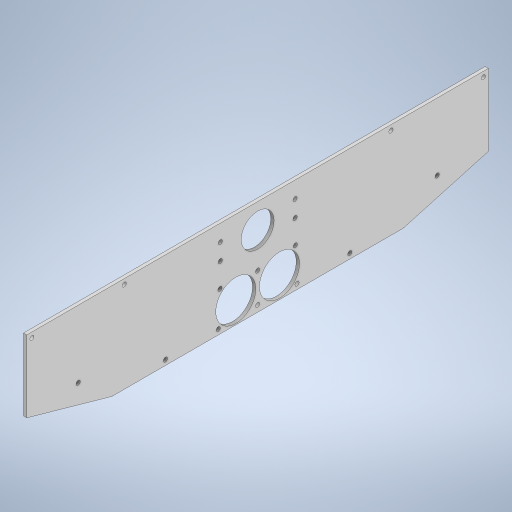
# Autodesk Inventor part: insideChassiPlate2.0
Saved by Autodesk Inventor 2023 (Build 270158000, 158)
## iProperties
Created: 2022-09-08
Part Number: insideChassiPlate2.0
Material: Generic
Document SubType Name: Modeling
Designer: deli
Density: 1 g/cm^3
Appearance: Default
Author: deli
Autodesk Inventor part; units mm, degrees
ref_plane "YZ Plane" through (0, 0, 0) normal (1, 0, 0) x (0, 1, 0)
ref_plane "XZ Plane" through (0, 0, 0) normal (0, 1, 0) x (-1, 0, 0)
ref_plane "XY Plane" through (0, 0, 0) normal (0, 0, 1) x (1, 0, 0)
sketch "Sketch1" plane through (0, 0, 0) normal (1, 0, 0) x (0, 1, 0)
  line L0 (-34.0027, 86.5738) -> (-104.0027, 86.5738) projected
  line L1 (-104.0027, 86.5738) -> (-127.2253, 4.3058) projected
  arc A0 (-127.2253, 4.3058) -> (-127.4133, 2.9475) centre (-122.4133, 2.9475) ccw projected
  line L2 (-127.4133, 2.9475) -> (-127.4133, -279.7999) projected
  arc A1 (-127.4133, -279.7999) -> (-127.2253, -281.1582) centre (-122.4133, -279.7999) ccw projected
  line L3 (-127.2253, -281.1582) -> (-104.0027, -363.4262) projected
  line L4 (-104.0027, -363.4262) -> (-34.0027, -363.4262) projected
  line L5 (-34.0027, -363.4262) -> (-34.0027, -226.9762) projected
  line L6 (-34.0027, -226.9762) -> (230.9973, -226.9762) projected
  line L7 (230.9973, -226.9762) -> (230.9973, -201.5762) projected
  line L8 (230.9973, -201.5762) -> (-34.0027, -201.5762) projected
  line L9 (-34.0027, -201.5762) -> (-34.0027, 86.5738) projected
  circle A2 centre (-66.0027, -101.9662) radius 2 projected
  circle A3 centre (-122.4133, -228.31) radius 2 projected
  circle A4 centre (-122.4133, -48.5424) radius 2 projected
  circle A5 centre (-39.0027, -8.4262) radius 2 projected
  circle A6 centre (-39.0027, -358.4262) radius 2 projected
  circle A7 centre (-89.2685, -175.1441) radius 2 projected
  circle A8 centre (-99.4133, 36.5738) radius 2 projected
  circle A9 centre (-99.4133, -313.4262) radius 2 projected
  circle A10 centre (-106.6633, -117.135) radius 7 construction
  circle A11 centre (-106.6633, -159.7175) radius 7 construction
  circle A12 centre (-92.1807, -138.4262) radius 2 projected
  circle A13 centre (-121.1459, -138.4262) radius 2 projected
  circle A14 centre (-122.4133, -100.0323) radius 2 projected
  circle A15 centre (-122.4133, -176.8201) radius 2 projected
  circle A16 centre (-39.0027, 81.5738) radius 2 projected
  circle A17 centre (-89.2685, -101.7083) radius 2 projected
  circle A18 centre (-39.0027, -268.4262) radius 2 projected
  circle A19 centre (222.9973, -212.6887) radius 2 projected
  circle A20 centre (-58.0027, -138.4262) radius 16 projected
  circle A21 centre (-50.0027, -101.9662) radius 2 projected
  line L10 (-34.0027, -201.5762) -> (-34.0027, -226.9762)
  spline S0 degree 3 poles (-44.0027, -174.8862) (-44.0027, -175.0973) (-43.9693, -175.3071) (-43.8358, -175.7154) (-43.7344, -175.9104) (-43.4447, -176.2972) (-43.2452, -176.4757) (-42.7979, -176.7388) (-42.5566, -176.8247) (-42.0448, -176.9031) (-41.7788, -176.8911) (-41.2697, -176.7652) (-41.0313, -176.6538) (-40.6137, -176.3479) (-40.4377, -176.1576) (-40.1619, -175.7123) (-40.0681, -175.4594) (-39.9874, -174.9441) (-39.9964, -174.6875) (-40.1114, -174.1861) (-40.2182, -173.9465) (-40.5206, -173.5174) (-40.7149, -173.3332) (-41.1541, -173.0576) (-41.3924, -172.9648) (-41.9003, -172.8716) (-42.1657, -172.8756) (-42.6799, -172.9861) (-42.9235, -173.0914) (-43.3506, -173.3866) (-43.5314, -173.5713) (-43.8189, -174.0074) (-43.9197, -174.2567) (-44.0156, -174.7696) (-44.0141, -175.0274) (-43.9132, -175.5321) (-43.8136, -175.774) (-43.5242, -176.2111) (-43.3354, -176.401) (-42.9045, -176.6892) (-42.6692, -176.7888) (-42.1652, -176.8968) (-41.9006, -176.9007) (-41.3816, -176.8057) (-41.1326, -176.7065) (-40.6963, -176.422) (-40.511, -176.2427) (-40.2122, -175.816) (-40.1048, -175.5704) (-39.9938, -175.0601) (-39.9881, -174.801) (-40.0753, -174.2932) (-40.168, -174.0493) (-40.4445, -173.6047) (-40.6279, -173.4096) (-41.0506, -173.1092) (-41.2831, -173.003) (-41.7833, -172.8812) (-42.047, -172.8697) (-42.5675, -172.9494) (-42.819, -173.0412) (-43.2627, -173.3122) (-43.4527, -173.4853) (-43.7634, -173.9013) (-43.8782, -174.1427) (-44.0055, -174.6501) (-44.0192, -174.9106) (-43.9469, -175.4217) (-43.8618, -175.6674) (-43.5979, -176.122) (-43.4182, -176.3244) (-43.0011, -176.6377) (-42.7711, -176.7501) (-42.2746, -176.8847) (-42.012, -176.9031) (-41.4904, -176.8376) (-41.2366, -176.7526) (-40.7865, -176.4941) (-40.5923, -176.3268) (-40.2708, -175.9206) (-40.1496, -175.6833) (-40.0072, -175.1788) (-39.9861, -174.9169) (-40.0451, -174.403) (-40.1233, -174.1557) (-40.3739, -173.6953) (-40.5474, -173.4886) (-40.9581, -173.1613) (-41.189, -173.0411) (-41.6904, -172.8931) (-41.9568, -172.8693) (-42.4735, -172.9258) (-42.7193, -173.0017) (-43.1803, -173.2476) (-43.3886, -173.4196) (-43.7216, -173.8308) (-43.8448, -174.0644) (-43.9918, -174.5579) (-44.0174, -174.8122) (-43.9712, -175.3286) (-43.8952, -175.5854) (-43.6507, -176.0485) (-43.4868, -176.2516) (-43.0923, -176.5829) (-42.8659, -176.7085) (-42.3694, -176.8702) (-42.103, -176.9013) (-41.5836, -176.8584) (-41.3353, -176.7888) (-40.8699, -176.5556) (-40.659, -176.391) (-40.3152, -175.9912) (-40.185, -175.7606) (-40.0238, -175.2709) (-39.9911, -175.0175) (-40.0225, -174.5) (-40.0911, -174.2412) (-40.3226, -173.7707) (-40.4812, -173.5625) (-40.8661, -173.2209) (-41.0877, -173.0896) (-41.5789, -172.9136) (-41.8451, -172.8747) (-42.3669, -172.903) (-42.6178, -172.966) (-43.0878, -173.1857) (-43.3013, -173.3426) (-43.6561, -173.7305) (-43.7936, -173.9577) (-43.9695, -174.4435) (-44.0097, -174.6961) (-43.9934, -175.2144) (-43.9324, -175.4751) (-43.7145, -175.9528) (-43.5615, -176.166) (-43.1865, -176.5182) (-42.9696, -176.6553) (-42.4841, -176.8457) (-42.2183, -176.8924) (-41.6944, -176.8789) (-41.4411, -176.8229) (-40.9667, -176.6166) (-40.7505, -176.4673) (-40.385, -176.0915) (-40.2403, -175.8678) (-40.0496, -175.3861) (-40.002, -175.1343) (-40.0035, -174.6152) (-40.057, -174.353) (-40.2614, -173.8686) (-40.4087, -173.6505) (-40.7738, -173.2881) (-40.9862, -173.1452) (-41.4662, -172.941) (-41.7314, -172.8867) (-42.2569, -172.8858) (-42.5123, -172.9351) (-42.991, -173.1283) (-43.2096, -173.2706) (-43.5852, -173.6348) (-43.7367, -173.8549) (-43.9413, -174.3322) (-43.996, -174.5833) (-44.0086, -175.103) (-43.9622, -175.3667) (-43.7706, -175.8572) (-43.6287, -176.0797) (-43.2729, -176.4517) (-43.0646, -176.5999) (-42.593, -176.8155) (-42.3322, -176.8766) (-41.809, -176.8935) (-41.5515, -176.8517) (-41.0682, -176.673) (-40.8468, -176.5384) (-40.4604, -176.1869) (-40.3016, -175.9709) (-40.0818, -175.4987) (-40.0193, -175.2486) (-39.9914, -174.7284) (-40.03, -174.4632) (-40.2076, -173.9663) (-40.3435, -173.7392) (-40.6892, -173.3569) (-40.8932, -173.2031) (-41.3584, -172.9744) (-41.6173, -172.9059) (-42.1406, -172.8742) (-42.3998, -172.909) (-42.8872, -173.0743) (-43.1112, -173.202) (-43.5072, -173.5418) (-43.6726, -173.7538) (-43.9062, -174.221) (-43.9757, -174.47) (-44.0174, -174.9874) (-43.9867, -175.2511) (-43.8249, -175.7515) (-43.6955, -175.9833) (-43.3606, -176.3764) (-43.161, -176.5362) (-42.7026, -176.7785) (-42.4458, -176.8544) (-41.923, -176.9014) (-41.6622, -176.8741) (-41.1706, -176.7226) (-40.9439, -176.6019) (-40.5382, -176.2741) (-40.3662, -176.0664) (-40.1187, -175.6048) (-40.0421, -175.3571) (-39.9863, -174.8425) (-40.0091, -174.5803) (-40.155, -174.0766) (-40.2778, -173.8403) (-40.6017, -173.4365) (-40.7969, -173.2705) (-41.2486, -173.015) (-41.5029, -172.9316) (-42.0248, -172.8694) (-42.2871, -172.8895) (-42.7828, -173.0272) (-43.0121, -173.1411) (-43.4272, -173.457) (-43.6055, -173.6603) (-43.8665, -174.1162) (-43.95, -174.3623) (-44.0194, -174.8741) (-44.004, -175.1349) (-43.8734, -175.6416) (-43.7572, -175.8821) (-43.4441, -176.296) (-43.2531, -176.4678) (-42.808, -176.736) (-42.556, -176.8264) (-42.0351, -176.9029) (-41.7717, -176.8899) (-41.2723, -176.7652) (-41.0404, -176.6577) (-40.6194, -176.3548) (-40.4371, -176.1586) (-40.1632, -175.7125) (-40.072, -175.4683) (-39.9876, -174.9599) (-39.9949, -174.7005) (-40.1089, -174.1907) (-40.2178, -173.9459) (-40.5188, -173.5212) (-40.705, -173.3431) (-41.1433, -173.0608) (-41.3933, -172.9628) (-41.9133, -172.8711) (-42.1778, -172.8767) (-42.6809, -172.9877) (-42.9156, -173.0888) (-43.3447, -173.3797) (-43.5324, -173.5707) (-43.8189, -174.0095) (-43.9171, -174.2518) (-44.0149, -174.7572) (-44.0149, -175.0153) (-43.9157, -175.5277) (-43.8135, -175.7762) (-43.5234, -176.2102) (-43.3417, -176.3938) (-42.9126, -176.6866) (-42.6678, -176.7907) (-42.1526, -176.8978) (-41.8873, -176.9001) (-41.3802, -176.8037) (-41.1426, -176.7095) (-40.7052, -176.4311) (-40.512, -176.2456) (-40.2124, -175.8148) (-40.1071, -175.5747) (-39.9952, -175.0726) (-39.9878, -174.8157) (-40.0718, -174.3009) (-40.167, -174.0488) (-40.4398, -173.6142) (-40.6083, -173.4315) (-40.9968, -173.1412) (-41.2121, -173.0337) (-41.4412, -172.9667) knots 0.000001 0.000001 0.000001 0.000001 0.063398 0.063398 0.128915 0.128915 0.208453 0.208453 0.284598 0.284598 0.36365 0.36365 0.441803 0.441803 0.518819 0.518819 0.598884 0.598884 0.675195 0.675195 0.753106 0.753106 0.832585 0.832585 0.908527 0.908527 0.987293 0.987293 1.06607 1.06607 1.142839 1.142839 1.222632 1.222632 1.299213 1.299213 1.376876 1.376876 1.456341 1.456341 1.532212 1.532212 1.610735 1.610735 1.690252 1.690252 1.766822 1.766822 1.846392 1.846392 1.923362 1.923362 2.000828 2.000828 2.080319 2.080319 2.156245 2.156245 2.234575 2.234575 2.31405 2.31405 2.390444 2.390444 2.469816 2.469816 2.547344 2.547344 2.624642 2.624642 2.705021 2.705021 2.781115 2.781115 2.859312 2.859312 2.938796 2.938796 3.01493 3.01493 3.093973 3.093973 3.171944 3.171944 3.248946 3.248946 3.329001 3.329001 3.406279 3.406279 3.485634 3.485634 3.562005 3.562005 3.642108 3.642108 3.720394 3.720394 3.796227 3.796227 3.875634 3.875634 3.953058 3.953058 4.029875 4.029875 4.109405 4.109405 4.185934 4.185934 4.265232 4.265232 4.34372 4.34372 4.419521 4.419521 4.498908 4.498908 4.576539 4.576539 4.652987 4.652987 4.732749 4.732749 4.809486 4.809486 4.888063 4.888063 4.966802 4.966802 5.042698 5.042698 5.122108 5.122108 5.199994 5.199994 5.276196 5.276196 5.356239 5.356239 5.433231 5.433231 5.51121 5.51121 5.590242 5.590242 5.666365 5.666365 5.745842 5.745842 5.824027 5.824027 5.900118 5.900118 5.980485 5.980485 6.057771 6.057771 6.135304 6.135304 6.214664 6.214664 6.291046 6.291046 6.370513 6.370513 6.448831 6.448831 6.524751 6.524751 6.604234 6.604234 6.681689 6.681689 6.758659 6.758659 6.838216 6.838216 6.914774 6.914774 6.994299 6.994299 7.072809 7.072809 7.148671 7.148671 7.228128 7.228128 7.305778 7.305778 7.382357 7.382357 7.462136 7.462136 7.538892 7.538892 7.617675 7.617675 7.696426 7.696426 7.772357 7.772357 7.851827 7.851827 7.929724 7.929724 8.00603 8.00603 8.08608 8.08608 8.163082 8.163082 8.241238 8.241238 8.320275 8.320275 8.396406 8.396406 8.475934 8.475934 8.554121 8.554121 8.630289 8.630289 8.710655 8.710655 8.787944 8.787944 8.865621 8.865621 8.944979 8.944979 9.021361 9.021361 9.100863 9.100863 9.179179 9.179179 9.255149 9.255149 9.334671 9.334671 9.412121 9.412121 9.489205 9.489205 9.568755 9.568755 9.645307 9.645307 9.725014 9.725014 9.803511 9.803511 9.879402 9.879402 9.958888 9.958888 10.036524 10.036524 10.113198 10.113198 10.192958 10.192958 10.269699 10.269699 10.348645 10.348645 10.427375 10.427375 10.503309 10.503309 10.582801 10.582801 10.660674 10.660674 10.737051 10.737051 10.817073 10.817073 10.890944 10.890944 10.962515 10.962515 10.962515 10.962515 projected
  spline S1 degree 3 poles (-76.0027, -174.8862) (-76.0027, -175.0973) (-75.9693, -175.3071) (-75.8358, -175.7154) (-75.7344, -175.9104) (-75.4447, -176.2972) (-75.2452, -176.4757) (-74.7979, -176.7388) (-74.5566, -176.8247) (-74.0448, -176.9031) (-73.7788, -176.8911) (-73.2697, -176.7652) (-73.0313, -176.6538) (-72.6137, -176.3479) (-72.4377, -176.1576) (-72.1619, -175.7123) (-72.0681, -175.4594) (-71.9874, -174.9441) (-71.9964, -174.6875) (-72.1114, -174.1861) (-72.2182, -173.9465) (-72.5206, -173.5174) (-72.7149, -173.3332) (-73.1541, -173.0576) (-73.3924, -172.9648) (-73.9003, -172.8716) (-74.1657, -172.8756) (-74.6799, -172.9861) (-74.9235, -173.0914) (-75.3506, -173.3866) (-75.5314, -173.5713) (-75.8189, -174.0074) (-75.9197, -174.2567) (-76.0156, -174.7696) (-76.0141, -175.0274) (-75.9132, -175.5321) (-75.8136, -175.774) (-75.5242, -176.2111) (-75.3354, -176.401) (-74.9045, -176.6892) (-74.6692, -176.7888) (-74.1652, -176.8968) (-73.9006, -176.9007) (-73.3816, -176.8057) (-73.1326, -176.7065) (-72.6963, -176.422) (-72.511, -176.2427) (-72.2122, -175.816) (-72.1048, -175.5704) (-71.9938, -175.0601) (-71.9881, -174.801) (-72.0753, -174.2932) (-72.168, -174.0493) (-72.4445, -173.6047) (-72.6279, -173.4096) (-73.0506, -173.1092) (-73.2831, -173.003) (-73.7833, -172.8812) (-74.047, -172.8697) (-74.5675, -172.9494) (-74.819, -173.0412) (-75.2627, -173.3122) (-75.4527, -173.4853) (-75.7634, -173.9013) (-75.8782, -174.1427) (-76.0055, -174.6501) (-76.0192, -174.9106) (-75.9469, -175.4217) (-75.8618, -175.6674) (-75.5979, -176.122) (-75.4182, -176.3244) (-75.0011, -176.6377) (-74.7711, -176.7501) (-74.2746, -176.8847) (-74.012, -176.9031) (-73.4904, -176.8376) (-73.2366, -176.7526) (-72.7865, -176.4941) (-72.5923, -176.3268) (-72.2708, -175.9206) (-72.1496, -175.6833) (-72.0072, -175.1788) (-71.9861, -174.9169) (-72.0451, -174.403) (-72.1233, -174.1557) (-72.3739, -173.6953) (-72.5474, -173.4886) (-72.9581, -173.1613) (-73.189, -173.0411) (-73.6904, -172.8931) (-73.9568, -172.8693) (-74.4735, -172.9258) (-74.7193, -173.0017) (-75.1803, -173.2476) (-75.3886, -173.4196) (-75.7216, -173.8308) (-75.8448, -174.0644) (-75.9918, -174.5579) (-76.0174, -174.8122) (-75.9712, -175.3286) (-75.8952, -175.5854) (-75.6507, -176.0485) (-75.4868, -176.2516) (-75.0923, -176.5829) (-74.8659, -176.7085) (-74.3694, -176.8702) (-74.103, -176.9013) (-73.5836, -176.8584) (-73.3353, -176.7888) (-72.8699, -176.5556) (-72.659, -176.391) (-72.3152, -175.9912) (-72.185, -175.7606) (-72.0238, -175.2709) (-71.9911, -175.0175) (-72.0225, -174.5) (-72.0911, -174.2412) (-72.3226, -173.7707) (-72.4812, -173.5625) (-72.8661, -173.2209) (-73.0877, -173.0896) (-73.5789, -172.9136) (-73.8451, -172.8747) (-74.3669, -172.903) (-74.6178, -172.966) (-75.0878, -173.1857) (-75.3013, -173.3426) (-75.6561, -173.7305) (-75.7936, -173.9577) (-75.9695, -174.4435) (-76.0097, -174.6961) (-75.9934, -175.2144) (-75.9324, -175.4751) (-75.7145, -175.9528) (-75.5615, -176.166) (-75.1865, -176.5182) (-74.9696, -176.6553) (-74.4841, -176.8457) (-74.2183, -176.8924) (-73.6944, -176.8789) (-73.4411, -176.8229) (-72.9667, -176.6166) (-72.7505, -176.4673) (-72.385, -176.0915) (-72.2403, -175.8678) (-72.0496, -175.3861) (-72.002, -175.1343) (-72.0035, -174.6152) (-72.057, -174.353) (-72.2614, -173.8686) (-72.4087, -173.6505) (-72.7738, -173.2881) (-72.9862, -173.1452) (-73.4662, -172.941) (-73.7314, -172.8867) (-74.2569, -172.8858) (-74.5123, -172.9351) (-74.991, -173.1283) (-75.2096, -173.2706) (-75.5852, -173.6348) (-75.7367, -173.8549) (-75.9413, -174.3322) (-75.996, -174.5833) (-76.0086, -175.103) (-75.9622, -175.3667) (-75.7706, -175.8572) (-75.6287, -176.0797) (-75.2729, -176.4517) (-75.0646, -176.5999) (-74.593, -176.8155) (-74.3322, -176.8766) (-73.809, -176.8935) (-73.5515, -176.8517) (-73.0682, -176.673) (-72.8468, -176.5384) (-72.4604, -176.1869) (-72.3016, -175.9709) (-72.0818, -175.4987) (-72.0193, -175.2486) (-71.9914, -174.7284) (-72.03, -174.4632) (-72.2076, -173.9663) (-72.3435, -173.7392) (-72.6892, -173.3569) (-72.8932, -173.2031) (-73.3584, -172.9744) (-73.6173, -172.9059) (-74.1406, -172.8742) (-74.3998, -172.909) (-74.8872, -173.0743) (-75.1112, -173.202) (-75.5072, -173.5418) (-75.6726, -173.7538) (-75.9062, -174.221) (-75.9757, -174.47) (-76.0174, -174.9874) (-75.9867, -175.2511) (-75.8249, -175.7515) (-75.6955, -175.9833) (-75.3606, -176.3764) (-75.161, -176.5362) (-74.7026, -176.7785) (-74.4458, -176.8544) (-73.923, -176.9014) (-73.6622, -176.8741) (-73.1706, -176.7226) (-72.9439, -176.6019) (-72.5382, -176.2741) (-72.3662, -176.0664) (-72.1187, -175.6048) (-72.0421, -175.3571) (-71.9863, -174.8425) (-72.0091, -174.5803) (-72.155, -174.0766) (-72.2778, -173.8403) (-72.6017, -173.4365) (-72.7969, -173.2705) (-73.2486, -173.015) (-73.5029, -172.9316) (-74.0248, -172.8694) (-74.2871, -172.8895) (-74.7828, -173.0272) (-75.0121, -173.1411) (-75.4272, -173.457) (-75.6055, -173.6603) (-75.8665, -174.1162) (-75.95, -174.3623) (-76.0194, -174.8741) (-76.004, -175.1349) (-75.8734, -175.6416) (-75.7572, -175.8821) (-75.4441, -176.296) (-75.2531, -176.4678) (-74.808, -176.736) (-74.556, -176.8264) (-74.0351, -176.9029) (-73.7717, -176.8899) (-73.2723, -176.7652) (-73.0404, -176.6577) (-72.6194, -176.3548) (-72.4371, -176.1586) (-72.1632, -175.7125) (-72.072, -175.4683) (-71.9876, -174.9599) (-71.9949, -174.7005) (-72.1089, -174.1907) (-72.2178, -173.9459) (-72.5188, -173.5212) (-72.705, -173.3431) (-73.1433, -173.0608) (-73.3933, -172.9628) (-73.9133, -172.8711) (-74.1778, -172.8767) (-74.6809, -172.9877) (-74.9156, -173.0888) (-75.3447, -173.3797) (-75.5324, -173.5707) (-75.8189, -174.0095) (-75.9171, -174.2518) (-76.0149, -174.7572) (-76.0149, -175.0153) (-75.9157, -175.5277) (-75.8135, -175.7762) (-75.5234, -176.2102) (-75.3417, -176.3938) (-74.9126, -176.6866) (-74.6678, -176.7907) (-74.1526, -176.8978) (-73.8873, -176.9001) (-73.3802, -176.8037) (-73.1426, -176.7095) (-72.7052, -176.4311) (-72.512, -176.2456) (-72.2124, -175.8148) (-72.1071, -175.5747) (-71.9952, -175.0726) (-71.9878, -174.8157) (-72.0718, -174.3009) (-72.167, -174.0488) (-72.4398, -173.6142) (-72.6083, -173.4315) (-72.9968, -173.1412) (-73.2121, -173.0337) (-73.4412, -172.9667) knots 0.000001 0.000001 0.000001 0.000001 0.063398 0.063398 0.128915 0.128915 0.208453 0.208453 0.284598 0.284598 0.36365 0.36365 0.441803 0.441803 0.518819 0.518819 0.598884 0.598884 0.675195 0.675195 0.753106 0.753106 0.832585 0.832585 0.908527 0.908527 0.987293 0.987293 1.06607 1.06607 1.142839 1.142839 1.222632 1.222632 1.299213 1.299213 1.376876 1.376876 1.456341 1.456341 1.532212 1.532212 1.610735 1.610735 1.690252 1.690252 1.766822 1.766822 1.846392 1.846392 1.923362 1.923362 2.000828 2.000828 2.080319 2.080319 2.156245 2.156245 2.234575 2.234575 2.31405 2.31405 2.390444 2.390444 2.469816 2.469816 2.547344 2.547344 2.624642 2.624642 2.705021 2.705021 2.781115 2.781115 2.859312 2.859312 2.938796 2.938796 3.01493 3.01493 3.093973 3.093973 3.171944 3.171944 3.248946 3.248946 3.329001 3.329001 3.406279 3.406279 3.485634 3.485634 3.562005 3.562005 3.642108 3.642108 3.720394 3.720394 3.796227 3.796227 3.875634 3.875634 3.953058 3.953058 4.029875 4.029875 4.109405 4.109405 4.185934 4.185934 4.265232 4.265232 4.34372 4.34372 4.419521 4.419521 4.498908 4.498908 4.576539 4.576539 4.652987 4.652987 4.732749 4.732749 4.809486 4.809486 4.888063 4.888063 4.966802 4.966802 5.042698 5.042698 5.122108 5.122108 5.199994 5.199994 5.276196 5.276196 5.356239 5.356239 5.433231 5.433231 5.51121 5.51121 5.590242 5.590242 5.666365 5.666365 5.745842 5.745842 5.824027 5.824027 5.900118 5.900118 5.980485 5.980485 6.057771 6.057771 6.135304 6.135304 6.214664 6.214664 6.291046 6.291046 6.370513 6.370513 6.448831 6.448831 6.524751 6.524751 6.604234 6.604234 6.681689 6.681689 6.758659 6.758659 6.838216 6.838216 6.914774 6.914774 6.994299 6.994299 7.072809 7.072809 7.148671 7.148671 7.228128 7.228128 7.305778 7.305778 7.382357 7.382357 7.462136 7.462136 7.538892 7.538892 7.617675 7.617675 7.696426 7.696426 7.772357 7.772357 7.851827 7.851827 7.929724 7.929724 8.00603 8.00603 8.08608 8.08608 8.163082 8.163082 8.241238 8.241238 8.320275 8.320275 8.396406 8.396406 8.475934 8.475934 8.554121 8.554121 8.630289 8.630289 8.710655 8.710655 8.787944 8.787944 8.865621 8.865621 8.944979 8.944979 9.021361 9.021361 9.100863 9.100863 9.179179 9.179179 9.255149 9.255149 9.334671 9.334671 9.412121 9.412121 9.489205 9.489205 9.568755 9.568755 9.645307 9.645307 9.725014 9.725014 9.803511 9.803511 9.879402 9.879402 9.958888 9.958888 10.036524 10.036524 10.113198 10.113198 10.192958 10.192958 10.269699 10.269699 10.348645 10.348645 10.427375 10.427375 10.503309 10.503309 10.582801 10.582801 10.660674 10.660674 10.737051 10.737051 10.817073 10.817073 10.890944 10.890944 10.962515 10.962515 10.962515 10.962515 projected
  circle A22 centre (-50.0027, -174.8862) radius 2 projected
  circle A23 centre (-66.0027, -174.8862) radius 2 projected
  circle A24 centre (-66.0027, -174.8862) radius 2
  circle A25 centre (-50.0027, -174.8862) radius 2
  line L11 (-50.0027, -101.9662) -> (-66.0027, -101.9662) construction
  line L12 (-66.0027, -101.9662) -> (-66.0027, -174.8862) construction
  line L13 (-66.0027, -174.8862) -> (-50.0027, -174.8862) construction
  line L14 (-50.0027, -174.8862) -> (-50.0027, -101.9662) construction
  circle A26 centre (-106.6633, -117.135) radius 19.5
  circle A27 centre (-106.6633, -159.7175) radius 19.5
  dimension "d6" = 4
  dimension "d7" = 4
  dimension "d8" = 39
  dimension "d9" = 39
  constraints: 10 end point, 4 centre point, 4 coincident, 2 parallel, 1 horizontal, 1 perpendicular, 1 vertical
  measures "d6" diameter of A24
  measures "d7" diameter of A25
  measures "d8" diameter of A26
  measures "d9" diameter of A27
extrude "Extrusion1" add sketch "Sketch1" along normal blind 3.175 contours L9 L10 L5 L4 L3 A1 L2 A0 L1 L0
body "Solid1"
